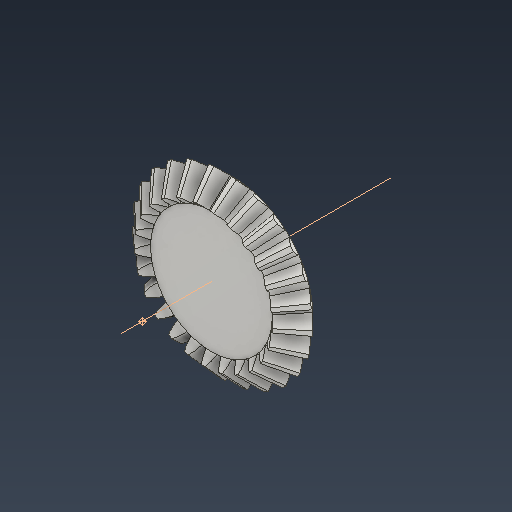
# Autodesk Inventor part: Коническая зубчатая передача2
Saved by Autodesk Inventor 2026 (Build 300175000, 175)
## iProperties
Created: 2026-01-11
Part Number: Коническая зубчатая передача2
Material: Steel, Mild
Document SubType Name: Modeling
Designer: GameHD
Categories: <?xml version="1.0" encoding="UTF-16"?> <MemberInstance><Categories><FamilyTemplate><FamilyTemplateParameter ValueType="xs:double" Id="1" ObjectReferenceKey="da_z" ObjectType="kUserParameterObject"/><FamilyTemplateParameter ValueType="xs:double" Id="2" ObjectReferenceKey="da_b" ObjectType="kUserParameterObject"/><FamilyTemplateParameter ValueType="xs:double" Id="3" ObjectReferenceKey="da_beta" ObjectType="kUserParameterObject"/><FamilyTemplateParameter ValueType="xs:double" Id="4" ObjectReferenceKey="da_dae" ObjectType="kUserParameterObject"/><FamilyTemplateParameter ValueType="xs:double" Id="5" ObjectReferenceKey="da_ve" ObjectType="kUserParameterObject"/><FamilyTemplateParameter ValueType="xs:double" Id="6" ObjectReferenceKey="da_omega" ObjectType="kUserParameterObject"/><FamilyTemplateParameter ValueType="xs:string" Id="7" ObjectReferenceKey="EAIAABAAAAAAHwAAAAAAAIAAAAAAAAAA" ObjectType="83914240" SubObjectId="SurfaceGeometry"/></FamilyTemplate><ParamToTemplateMap><ParamToTemplate CategoryParameter="//CategoryParameter[@InternalName='046C89C9-8512-4d59-83FE-43B91F4F132A']" TemplateParameter="1"/><ParamToTemplate CategoryParameter="//CategoryParameter[@InternalName='2552DF32-E462-4b46-AEBF-C6C7768E72AC']" TemplateParameter="2"/><ParamToTemplate CategoryParameter="//CategoryParameter[@InternalName='C9EE641D-15FC-4fae-A226-E94C4372FDD7']" TemplateParameter="3"/><ParamToTemplate><ParamToTemplate CategoryParameter="//CategoryParameter[@InternalName='00B6519A-459B-49c7-AD84-2E56D39A5744']" ConstantValue="-0.000000"/></ParamToTemplate><ParamToTemplate><ParamToTemplate CategoryParameter="//CategoryParameter[@InternalName='04B31F0E-C7A6-4894-AA32-9629BEFACF47']" ConstantValue="1.000000"/></ParamToTemplate><ParamToTemplate><ParamToTemplate CategoryParameter="//CategoryParameter[@InternalName='43CBEC2E-7847-49e7-A936-2F7889FCB2D9']" ConstantValue="0.200000"/></ParamToTemplate><ParamToTemplate><ParamToTemplate CategoryParameter="//CategoryParameter[@InternalName='B1EFC894-105D-4ebd-86BF-FA20ED196853']" ConstantValue="0.300000"/></ParamToTemplate><ParamToTemplate><ParamToTemplate CategoryParameter="//CategoryParameter[@InternalName='51175063-3D10-4879-93E8-6246FE8B403D']" ConstantValue="2060000000.000000"/></ParamToTemplate><ParamToTemplate><ParamToTemplate CategoryParameter="//CategoryParameter[@InternalName='A3A52E27-4454-46a9-B0BD-C932399B70AF']" ConstantValue="0.300000"/></ParamToTemplate><ParamToTemplate CategoryParameter="//CategoryParameter[@InternalName='2A200944-5A8C-41ca-B96E-8520D2E510F1']" TemplateParameter="4"/><ParamToTemplate><ParamToTemplate CategoryParameter="//CategoryParameter[@InternalName='1A637F62-92C8-44bc-B81F-10802510B579']" ConstantValue="2.013852"/></ParamToTemplate><ParamToTemplate CategoryParameter="//CategoryParameter[@InternalName='B52DD4BE-6863-48fb-BF58-89EF6F9EC65C']" TemplateParameter="5"/><ParamToTemplate><ParamToTemplate CategoryParameter="//CategoryParameter[@InternalName='3956BFF2-84D2-457d-93C2-9B0613DEBA67']" ConstantValue="0.899104"/></ParamToTemplate><ParamToTemplate CategoryParameter="//CategoryParameter[@InternalName='739CFA02-461B-4bf8-8049-181FCAD8B28F']" TemplateParameter="6"/><ParamToTemplate><ParamToTemplate CategoryParameter="//CategoryParameter[@InternalName='A27E999F-E2CE-4481-8A2A-EBF499C4C3C5']" ConstantValue="-0.000000"/></ParamToTemplate><ParamToTemplate><ParamToTemplate CategoryParameter="//CategoryParameter[@InternalName='9E1B4470-B2D3-4ff1-B813-535BB4CDF51A']" ConstantValue="3520000.000000"/></ParamToTemplate><ParamToTemplate><ParamToTemplate CategoryParameter="//CategoryParameter[@InternalName='F8452263-BFF6-458c-9FB1-07C4B99E95CD']" ConstantValue="11400000.000000"/></ParamToTemplate><ParamToTemplate><ParamToTemplate CategoryParameter="//CategoryParameter[@InternalName='3E3BB259-FD49-497f-8171-6EBC954A3479']" ConstantValue="2.000000"/></ParamToTemplate><ParamToTemplate CategoryParameter="//CategoryParameter[@InternalName='27C3BAF2-7550-4e4b-AE2C-0DB134B7D9B7']" TemplateParameter="7"/></ParamToTemplateMap><Category DisplayName="Gear" InternalName="DC85795E-93AB-48d5-8EEE-5A27447B64BD" Mnemonic="Gear"><CategoryParameter DisplayName="z" InternalName="046C89C9-8512-4d59-83FE-43B91F4F132A" Mnemonic="z"/><CategoryParameter DisplayName="b" InternalName="2552DF32-E462-4b46-AEBF-C6C7768E72AC" Mnemonic="b"/><CategoryParameter DisplayName="||b|" InternalName="C9EE641D-15FC-4fae-A226-E94C4372FDD7" Mnemonic="beta"/><CategoryParameter DisplayName="x" InternalName="00B6519A-459B-49c7-AD84-2E56D39A5744" Mnemonic="x"/><CategoryParameter DisplayName="a*" InternalName="04B31F0E-C7A6-4894-AA32-9629BEFACF47" Mnemonic="a"/><CategoryParameter DisplayName="c*" InternalName="43CBEC2E-7847-49e7-A936-2F7889FCB2D9" Mnemonic="c"/><CategoryParameter DisplayName="r|.f|*" InternalName="B1EFC894-105D-4ebd-86BF-FA20ED196853" Mnemonic="rf"/><CategoryParameter DisplayName="E" InternalName="51175063-3D10-4879-93E8-6246FE8B403D" Mnemonic="E"/><CategoryParameter DisplayName="||m|" InternalName="A3A52E27-4454-46a9-B0BD-C932399B70AF" Mnemonic="mi"/><Category DisplayName="BevelGear" InternalName="0C98F69A-0C2B-4791-B2FE-7691BB227E77" Mnemonic="BevelGear"><CategoryParameter DisplayName="d|.ae|" InternalName="2A200944-5A8C-41ca-B96E-8520D2E510F1" Mnemonic="dae"/><CategoryParameter DisplayName="d|.ai|" InternalName="1A637F62-92C8-44bc-B81F-10802510B579" Mnemonic="dai"/><CategoryParameter DisplayName="J|.e|" InternalName="B52DD4BE-6863-48fb-BF58-89EF6F9EC65C" Mnemonic="ve"/><CategoryParameter DisplayName="J|.i|" InternalName="3956BFF2-84D2-457d-93C2-9B0613DEBA67" Mnemonic="vi"/><CategoryParameter DisplayName="||S|" InternalName="739CFA02-461B-4bf8-8049-181FCAD8B28F" Mnemonic="omega"/><CategoryParameter DisplayName="x|.t|" InternalName="A27E999F-E2CE-4481-8A2A-EBF499C4C3C5" Mnemonic="xt"/><CategoryParameter DisplayName="||s||.Flim|" InternalName="9E1B4470-B2D3-4ff1-B813-535BB4CDF51A" Mnemonic="sFlim"/><CategoryParameter DisplayName="||s||.Hlim|" InternalName="F8452263-BFF6-458c-9FB1-07C4B99E95CD" Mnemonic="sHlim"/><CategoryParameter DisplayName="тип" InternalName="3E3BB259-FD49-497f-8171-6EBC954A3479" Mnemonic="type"/><CategoryParameter DisplayName="PitchDiameter" InternalName="27C3BAF2-7550-4e4b-AE2C-0DB134B7D9B7" Mnemonic="IDS_PITCHDIAM"/></Category></Category></Categories></MemberInstance>
Mass: 60.9118 g
Surface Area: 34.3074 cm^2
Volume: 7.7496 cm^3
Density: 7.86 g/cm^3
Appearance: Steel
CustomPartVersion: 1
Author: GameHD
Autodesk Inventor part; units mm, degrees
ref_plane "Плоскость сетки 2" through (0, 0, 0) normal (0.9921147, 0.1253332, 0) x (0, 0, 1)
sketch "Эскиз тела зубьев" plane through (0, 0, 0) normal (1, 0, 0) x (0, 1, 0)
  line L0 (0, 0) -> (11.651472, -13.348528) construction
  line L1 (11.651472, -13.348528) -> (13.207107, -11.792893)
  line L2 (13.207107, -11.792893) -> (0, 0) construction
  line L3 (12.5, -12.5) -> (0, 0) construction
  line L4 (8.883223, -10.17708) -> (10.069258, -8.991045)
  line L5 (11.651472, -13.348528) -> (8.883223, -10.17708)
  line L6 (13.207107, -11.792893) -> (10.069258, -8.991045)
  line L7 (0, -14.818234) -> (0, 2.469706)
  line L8 (0, -12.5) -> (13.207107, -12.5) construction
  dimension "d0" = 25
  dimension "d1" = 23.30294
  dimension "d2" = 26.41421
  dimension "d3" = 4.2
  dimension "d4" = 11.79289
  constraints: 16 end point, 4 point on line, 3 perpendicular, 2 collinear, 1 horizontal alignment, 1 vertical alignment
  measures "d0" diameter of L3.start L7
  measures "d1" diameter of L0.end L7
  measures "d2" diameter of L1.end L7
  measures "d3" distance between parallel lines of L1 L4
  measures "d4" vertical distance of L1.end L0.start
revolve "Тело зубьев" add sketch "Эскиз тела зубьев" angle 360 about axis through (0, 0, 0) along (0, 0, 1)
ref_plane "Плоскость зуба" through (0, 12.5, -12.5) normal (0, -0.7071068, 0.7071068) x (1, 0, 0)
sketch "Создать эскиз" plane through (0, 12.5, -12.5) normal (0, -0.7071068, 0.7071068) x (1, 0, 0)
  line L0 (0, -19.850453) -> (0, 5.258529)
  arc A0 (-0.383202, -1.464) -> (-1.754107, 1.580279) centre (-6.691351, -2.473882) ccw
  arc A1 (1.754107, 1.580279) -> (0.383202, -1.464) centre (6.691351, -2.473882) ccw
  line L1 (-0.383202, -1.464) -> (0.383202, -1.464)
  arc A2 (1.754107, 1.580279) -> (-1.754107, 1.580279) centre (0, -17.67767) ccw
  dimension "d7" = 6.38847
  dimension "d8" = 6.69135
  dimension "d9" = 15.20379
  dimension "d57" = 19.33767
  dimension "d58" = 16.21367
  constraints: 6 point on circle, 3 centre point, 3 symmetric about line, 2 end point, 1 coincident, 1 perpendicular, 1 other
  measures "d7" radius of A0
  measures "d8" horizontal distance of point (0, -17.678) A0.centre
  measures "d9" vertical distance of point (0, -17.678) A0.centre
  measures "d57" radius of A2
  measures "d58" distance from line of A2.centre L1
ref_plane "Конечная плоскость" through (0, 9.45237, -9.45237) normal (0, -0.7071068, 0.7071068) x (1, 0, 0)
sketch "Конечный эскиз" plane through (0, 9.45237, -9.45237) normal (0, -0.7071068, 0.7071068) x (1, 0, 0)
  line L0 (0, -11.78258) -> (0, 3.121291)
  arc A0 (-0.289774, -1.107062) -> (-1.326437, 1.19499) centre (-5.05993, -1.870724) ccw
  arc A1 (1.326437, 1.19499) -> (0.289774, -1.107062) centre (5.05993, -1.870724) ccw
  line L1 (-0.289774, -1.107062) -> (0.289774, -1.107062)
  arc A2 (1.326437, 1.19499) -> (-1.326437, 1.19499) centre (0, -13.36767) ccw
  dimension "d12" = 4.8309
  dimension "d15" = 5.05993
  dimension "d16" = 11.49695
  dimension "d59" = 14.62294
  dimension "d60" = 12.26061
  constraints: 6 point on circle, 3 centre point, 3 symmetric about line, 2 end point, 1 coincident, 1 other
  measures "d12" radius of A0
  measures "d15" horizontal distance of A0.centre point (0, -13.368)
  measures "d16" vertical distance of A0.centre point (0, -13.368)
  measures "d59" radius of A2
  measures "d60" distance from line of A2.centre L1
loft "Loft" cut profiles "Создать эскиз", "Конечный эскиз"
pattern_circular "Circular Pattern" count 25 over 360 about axis through (0, 0, 0) along (0, 0, 1) of "Loft"
sketch3d "3D эскиз: справа"
ref_plane "Конечная плоскость: справа" through (-4.267202, 8.434351, -9.45237) normal (0.3192181, -0.6309515, 0.7071068) x (0.8923002, 0.4514426, 0)
sketch "Конечный эскиз: справа" plane through (-4.267202, 8.434351, -9.45237) normal (0.3192181, -0.6309515, 0.7071068) x (0.8923002, 0.4514426, 0)
  arc A0 (-0.289774, -1.107062) -> (-1.326437, 1.19499) centre (-5.05993, -1.870724) ccw
  line L0 (0, -19.189733) -> (0, 6.81423)
  arc A1 (1.326437, 1.19499) -> (0.289774, -1.107062) centre (5.05993, -1.870724) ccw
  line L1 (-0.289774, -1.107062) -> (0.289774, -1.107062)
  arc A2 (1.326437, 1.19499) -> (-1.326437, 1.19499) centre (0, -13.36767) ccw
  dimension "d70" = 5.05993
  dimension "d71" = 11.49695
  dimension "d72" = 4.8309
  dimension "d73" = 12.26061
  dimension "d74" = 14.62294
  constraints: 6 point on circle, 3 centre point, 3 symmetric about line, 2 end point, 1 coincident, 1 perpendicular, 1 other
  measures "d70" horizontal distance of A2.centre A0.centre
  measures "d71" vertical distance of point (0, -13.368) A0.centre
  measures "d72" radius of A0
  measures "d73" distance from line of point (0, -13.368) L1
  measures "d74" radius of A2
feature "Лофт: справа" [suppressed]
pattern_circular "Круговой массив: справа" [suppressed]
sketch3d "3D эскиз: слева"
ref_plane "Конечная плоскость: cлева" through (4.031972, 8.434351, -9.147349) normal (-0.3082703, -0.6448607, 0.699374) x (0.9022112, -0.4312946, 0)
sketch "Конечный эскиз: слева" plane through (4.031972, 8.434351, -9.147349) normal (-0.3082703, -0.6448607, 0.699374) x (0.9022112, -0.4312946, 0)
  line L0 (0, -21.981289) -> (0, 9.381315)
  arc A0 (-0.289774, -1.251666) -> (-1.326437, 1.050386) centre (-5.05993, -2.015328) ccw
  arc A1 (1.326437, 1.050386) -> (0.289774, -1.251666) centre (5.05993, -2.015328) ccw
  line L1 (-0.289774, -1.251666) -> (0.289774, -1.251666)
  ellipse E0 centre (0, -6.426402) end of major axis (10.069258, -6.426402) minor radius 7.042178
  arc A2 (1.326437, 1.050386) -> (-1.326437, 1.050386) centre (0, -13.512274) ccw
  dimension "d56" = 7.04218
  dimension "d30" = 4.8309
  dimension "d31" = 5.05993
  dimension "d32" = 11.49695
  dimension "d61" = 14.62294
  dimension "d62" = 12.26061
  constraints: 6 point on circle, 3 centre point, 3 symmetric about line, 2 end point, 1 coincident, 2 other
  measures "d30" radius of A0
  measures "d31" horizontal distance of point (0, -13.512) A0.centre
  measures "d32" vertical distance of A0.centre point (0, -13.512)
  measures "d61" radius of A2
  measures "d62" distance from line of point (0, -13.512) L1
feature "Лофт: слева" [suppressed]
pattern_circular "Круговой массив: слева" [suppressed]
sketch "Эскиз тела" plane through (0, 0, 0) normal (1, 0, 0) x (0, 1, 0)
  line L0 (0, -13.335593) -> (0, -6.426139)
  line L1 (11.651472, -13.348528) -> (8.883223, -10.17708)
  line L2 (8.883223, -10.17708) -> (0, -10.17708)
  line L3 (11.651472, -13.348528) -> (0, -13.348528)
  constraints: 4 end point, 2 perpendicular, 2 point on line
sketch "Эскиз тела outline for Фиксировать тело" plane through (0, 0, 0) normal (1, 0, 0) x (0, 1, 0)
  line L0 (0, -13.348528) -> (11.651472, -13.348528)
  line L1 (0, -10.17708) -> (0, -13.348528)
  line L2 (8.883223, -10.17708) -> (0, -10.17708)
  line L3 (11.651472, -13.348528) -> (8.883223, -10.17708)
revolve "Фиксировать тело" add sketch "Эскиз тела outline for Фиксировать тело" angle 360 about axis through (0, 0, 0) along (0, 0, 1)
sketch "Sketch6" plane through (0, 0, 0) normal (1, 0, 0) x (0, 1, 0)
  line L0 (12.5, -12.5) -> (0, 0) projected
  line L1 (0, -13.8) -> (0, 2.3) projected
surface revolve "Средний диаметр" sketch "Sketch6" angle 360 about axis through (0, 0, 0) along (0, 0, 1) shown no curves L0
equation "\"d0\" = da_de"
equation "\"d1\" = da_dfe"
equation "\"d2\" = da_dae"
equation "\"d3\" = da_b"
equation "\"d4\" = da_ve"
equation "\"d7\" = fd_rr"
equation "\"d8\" = fd_x"
equation "\"d9\" = fd_y"
equation "\"d57\" = 0.5 * fd_dva + 0.3 * da_he"
equation "\"d58\" = 0.5 * fd_dva - 1.12 * da_he"
equation "\"da_teethtype\" = 0"
equation "\"da_b\" = 4.2"
equation "\"da_de\" = 25"
equation "\"da_dae\" = 26.41421"
equation "\"da_dfe\" = 23.30294"
equation "\"da_le\" = 17.67767"
equation "\"da_omega\" = 90deg"
equation "\"da_beta\" = 0"
equation "\"da_delta\" = 45deg"
equation "\"da_alpha\" = 20deg"
equation "\"da_he\" = 2.2"
equation "\"da_ve\" = 11.79289"
equation "\"da_zv\" = 35.355339"
equation "\"fd_loft\" = da_b + 0.05 * da_he"
equation "\"fd_x\" = fd_x1 + fd_x2"
equation "\"fd_y\" = fd_y1 - fd_y2"
equation "\"fd_dd\" = fd_dva - 0.8 * da_he"
equation "\"da_dvw\" = 35.35534"
equation "\"d11\" = fd_loft"
equation "\"da_dm\" = 22.03015"
equation "\"da_x\" = 0"
equation "\"da_m\" = 1"
equation "\"d50\" = da_omega"
equation "\"fd_rr\" = 6.388474"
equation "\"fd_dva\" = 37.355339"
equation "\"fd_x1\" = 0.793858"
equation "\"fd_x2\" = 5.897493"
equation "\"fd_y1\" = 17.659836"
equation "\"fd_y2\" = 2.456048"
body "Solid1"
body "Srf1"
